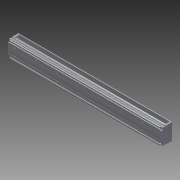
# Autodesk Inventor part: GL15N11060CASW' Body2
Saved by Autodesk Inventor 2011 SP1 (Build 150282100, 282)
## iProperties
Created: 2013-10-24
Part Number: GL15N11060CASW' Body2
Catalog Web Link: www.cadenas.de
Description: Type GL-N-body2-
Vendor: THK
Document SubType Name: Modeling
Designer: PARTuser1
Manufacturer: THK
Density: 1 g/cm^3
Category: PARTsolutions
Company: THK
Title: GL15N11060CASW' Body2
Author: Cadenas PARTsolutions
PSOL_IDENT_0: {$CADENAS_DATA\23d-libs\thk\actuator\type_gl_n\type_gl_n_f_na_1.prj},215 {VTYP=3D},{NB=GL15N11060CAS
PSOL_IDENT_1: W' Body2},{LINA=GL15N11060CASW' Body2},{NN=Type GL-N-body2},{DATE=29.11.2012 11:43:39},{GEOMDATE=29.
PSOL_IDENT_2: 11.2012 11:43:00},{VERSION=},{LINEID=10},{LINESUBID=-1},{WBVAR=L,C,LM,BSE,BSM,LML,BSL}  {NB=GL15N110
PSOL_IDENT_3: 60CASW' Body2},{LINA=GL15N11060CASW' Body2},{KT=DUMMY},{IDNR=},{MN=GL15N},{L=1060},{C=C},{LX=340,460
PSOL_IDENT_4: ,580,700,820,1060,1240,1420},{LM=SW},{VER=1},{DS=Ball screw kit},{BSE=A},{R=15.000},{NDM=2.000},{PCD
PSOL_IDENT_5: =23.000},{BSM=},{BSE1='A','A:inner diameter 30H7,M4,PCD46','B','B:inner diameter 50H7,M5,PCD70','C',
PSOL_IDENT_6: 'C:inner diameter 50H7,M4,PCD60','E','E:inner diameter 30H7,M3,PCD45','F','F:inner diameter 50H7,M4,
PSOL_IDENT_7: PCD70','G','G:inner diameter 34H7,M3,PCD48','H','H:inner diameter 36H7,M4,mounting aperture pitch 50
PSOL_IDENT_8: ','T'  , 'T:inner diameter 22,counter bore for M3 from rear,mounting pitch 31', 'U'  , 'U:inner diam
PSOL_IDENT_9: eter 38.1,M3.mounting pitch 47.14', 'W'  , 'W:inner diameter 40H7 ,M5,PCD63', 'Z'  , 'Z:inner diamet
PSOL_IDENT_10: er 60H7 ,M5,PCD75'},{SD=39},{SD1=27},{TL=126.000},{B=38.000},{TL1=160.000},{B1=45.000},{DS1=Bx},{LML
PSOL_IDENT_11: ='},{BSL=},{BSL1='', 'No mark:Not provided with QZ', 'Q', 'Q:Provided with QZ'},{N=6},{N1=4},{N2=6.0
PSOL_IDENT_12: 00},{N3=4},{BSM1='', 'No:Direct mounting', 'R1', 'R1:Right side motor wrap', 'R2'  , 'R2:Left side m
PSOL_IDENT_13: otor wrap', 'R3', 'R3:Bottom'}
CNS_NB: GL15N11060CASW' Body2
CNS_NBSYN: $MN.$VER.$L.$C.$BSE.$BSM.$LM.$LML.$BSL. Body2
CNS_LINA: GL15N11060CASW' Body2
CNS_MN: GL15N
CNS_L: 1060
CNS_C: Yes
CNS_LX: 340,460,580,700,820,1060,1240,1420
CNS_LM: SSR-XW (L-type table)
CNS_VER: 1
CNS_DS: Ball screw kit
CNS_BSE: A:inner diameter 30H7,M4,PCD46
CNS_R: 15.000
CNS_NDM: 2.000
CNS_PCD: 23.000
CNS_BSM: No:Direct mounting
CNS_BSE1: 'A','A:inner diameter 30H7,M4,PCD46','B','B:inner diameter 50H7,M5,PCD70','C','C:inner diameter 50H7,M4,PCD60','E','E:inner diameter 30H7,M3,PCD45','F','F:inner diameter 50H7,M4,PCD70','G','G:inner diameter 34H7,M3,PCD48','H','H:inner diameter 36H7,M4,mounting aperture pitch 50','T'  , 'T:inner diameter 22,counter bore for M3 from rear,mounting pitch 31', 'U'  , 'U:inner diameter 38.1,M3.mounting pitch 47.14', 'W'  , 'W:inner diameter 40H7 ,M5,PCD63', 'Z'  , 'Z:inner diameter 60H7 ,M5,PCD75'
CNS_SD: 39
CNS_SD1: 27
CNS_TL: 126.000
CNS_B: 38.000
CNS_TL1: 160.000
CNS_B1: 45.000
CNS_DS1: Bx
CNS_LML: No mark:Not provided with QZ
CNS_BSL: No mark:Not provided with QZ
CNS_BSL1: '', 'No mark:Not provided with QZ', 'Q', 'Q:Provided with QZ'
CNS_N: 6.000
CNS_N1: 4.000
CNS_N2: 6.000
CNS_N3: 4.000
CNS_BSM1: '', 'No:Direct mounting', 'R1', 'R1:Right side motor wrap', 'R2'  , 'R2:Left side motor wrap', 'R3', 'R3:Bottom'
SUPPLIER: THK
ARTICLENO: GL15N11060CASW' Body2
BOMINFO: GL15N11060CASW' Body2
CREATOR: CADENAS GmbH
Autodesk Inventor part; units mm, degrees
sketch "Sketch_1" plane through (0, 0, 0) normal (1, 0, 0) x (0, 1, 0)
  line L0 (18.1, 58) -> (12.47, 58)
  arc A0 (12.47, 58) -> (12, 57.53) centre (12.47, 57.53) ccw
  line L1 (12, 57.53) -> (12, 54.97)
  arc A1 (11.53, 54.5) -> (12, 54.97) centre (11.53, 54.97) ccw
  line L2 (11.53, 54.5) -> (6.47, 54.5)
  arc A2 (6, 54.97) -> (6.47, 54.5) centre (6.47, 54.97) ccw
  line L3 (6, 54.97) -> (6, 57.53)
  arc A3 (6, 57.53) -> (5.53, 58) centre (5.53, 57.53) ccw
  line L4 (5.53, 58) -> (3.14, 58)
  arc A4 (3.14, 58) -> (0, 54.86) centre (3.14, 54.86) ccw
  line L5 (0, 54.86) -> (0, 48.5)
  arc A5 (0, 48.5) -> (0.5, 48) centre (0.5, 48.5) ccw
  line L6 (0.5, 48) -> (3.5, 48)
  arc A6 (3.5, 48) -> (4, 48.5) centre (3.5, 48.5) ccw
  line L7 (4, 48.5) -> (4, 50)
  arc A7 (4.5, 50.5) -> (4, 50) centre (4.5, 50) ccw
  line L8 (4.5, 50.5) -> (8.5, 50.5)
  arc A8 (9, 50) -> (8.5, 50.5) centre (8.5, 50) ccw
  line L9 (9, 50) -> (9, 48.8)
  arc A9 (9, 48.8) -> (9.3, 48.5) centre (9.3, 48.8) ccw
  line L10 (9.3, 48.5) -> (9.7, 48.5)
  arc A10 (10, 48.2) -> (9.7, 48.5) centre (9.7, 48.2) ccw
  line L11 (10, 48.2) -> (10, 41.8)
  arc A11 (9.7, 41.5) -> (10, 41.8) centre (9.7, 41.8) ccw
  line L12 (9.7, 41.5) -> (9.3, 41.5)
  arc A12 (9.3, 41.5) -> (9, 41.2) centre (9.3, 41.2) ccw
  line L13 (9, 41.2) -> (9, 40)
  arc A13 (8.5, 39.5) -> (9, 40) centre (8.5, 40) ccw
  line L14 (8.5, 39.5) -> (4.5, 39.5)
  arc A14 (4, 40) -> (4.5, 39.5) centre (4.5, 40) ccw
  line L15 (4, 40) -> (4, 41.5)
  arc A15 (4, 41.5) -> (3.5, 42) centre (3.5, 41.5) ccw
  line L16 (3.5, 42) -> (0.5, 42)
  arc A16 (0.5, 42) -> (0, 41.5) centre (0.5, 41.5) ccw
  line L17 (0, 41.5) -> (0, 24)
  line L18 (0, 24) -> (0.531, 22.938)
  arc A17 (0.635, 22.4347) -> (0.531, 22.938) centre (-0.3634, 22.4908) ccw
  arc A18 (0.635, 22.4347) -> (0.635, -22.4347) centre (400.0054, 0) ccw
  arc A19 (0.531, -22.938) -> (0.635, -22.4347) centre (-0.3634, -22.4908) ccw
  line L19 (0.531, -22.938) -> (0, -24)
  line L20 (0, -24) -> (0, -41.5)
  arc A20 (0, -41.5) -> (0.5, -42) centre (0.5, -41.5) ccw
  line L21 (0.5, -42) -> (3.5, -42)
  arc A21 (3.5, -42) -> (4, -41.5) centre (3.5, -41.5) ccw
  line L22 (4, -41.5) -> (4, -40)
  arc A22 (4.5, -39.5) -> (4, -40) centre (4.5, -40) ccw
  line L23 (4.5, -39.5) -> (8.5, -39.5)
  arc A23 (9, -40) -> (8.5, -39.5) centre (8.5, -40) ccw
  line L24 (9, -40) -> (9, -41.2)
  arc A24 (9, -41.2) -> (9.3, -41.5) centre (9.3, -41.2) ccw
  line L25 (9.3, -41.5) -> (9.7, -41.5)
  arc A25 (10, -41.8) -> (9.7, -41.5) centre (9.7, -41.8) ccw
  line L26 (10, -41.8) -> (10, -48.2)
  arc A26 (9.7, -48.5) -> (10, -48.2) centre (9.7, -48.2) ccw
  line L27 (9.7, -48.5) -> (9.3, -48.5)
  arc A27 (9.3, -48.5) -> (9, -48.8) centre (9.3, -48.8) ccw
  line L28 (9, -48.8) -> (9, -50)
  arc A28 (8.5, -50.5) -> (9, -50) centre (8.5, -50) ccw
  line L29 (8.5, -50.5) -> (4.5, -50.5)
  arc A29 (4, -50) -> (4.5, -50.5) centre (4.5, -50) ccw
  line L30 (4, -50) -> (4, -48.5)
  arc A30 (4, -48.5) -> (3.5, -48) centre (3.5, -48.5) ccw
  line L31 (3.5, -48) -> (0.5, -48)
  arc A31 (0.5, -48) -> (0, -48.5) centre (0.5, -48.5) ccw
  line L32 (0, -48.5) -> (0, -54.86)
  arc A32 (0, -54.86) -> (3.14, -58) centre (3.14, -54.86) ccw
  line L33 (3.14, -58) -> (5.53, -58)
  arc A33 (5.53, -58) -> (6, -57.53) centre (5.53, -57.53) ccw
  line L34 (6, -57.53) -> (6, -54.97)
  arc A34 (6.47, -54.5) -> (6, -54.97) centre (6.47, -54.97) ccw
  line L35 (6.47, -54.5) -> (11.53, -54.5)
  arc A35 (12, -54.97) -> (11.53, -54.5) centre (11.53, -54.97) ccw
  line L36 (12, -54.97) -> (12, -57.53)
  arc A36 (12, -57.53) -> (12.47, -58) centre (12.47, -57.53) ccw
  line L37 (12.47, -58) -> (18.1, -58)
  line L38 (18.1, -58) -> (18.1, -57)
  line L39 (18.1, -57) -> (20.98, -57)
  arc A37 (20.98, -57) -> (21.45, -56.53) centre (20.98, -56.53) ccw
  line L40 (21.45, -56.53) -> (21.45, -55.97)
  arc A38 (21.45, -55.97) -> (20.98, -55.5) centre (20.98, -55.97) ccw
  line L41 (20.98, -55.5) -> (20.9, -55.5)
  arc A39 (20.7, -55.3) -> (20.9, -55.5) centre (20.9, -55.3) ccw
  line L42 (20.7, -55.3) -> (20.7, -53.3)
  arc A40 (21, -53) -> (20.7, -53.3) centre (21, -53.3) ccw
  line L43 (21, -53) -> (22, -53)
  arc A41 (22, -53) -> (22.2, -52.8) centre (22, -52.8) ccw
  arc A42 (22.5, -52.5) -> (22.2, -52.8) centre (22.5, -52.8) ccw
  line L44 (22.5, -52.5) -> (24.7, -52.5)
  arc A43 (25, -52.8) -> (24.7, -52.5) centre (24.7, -52.8) ccw
  arc A44 (25, -52.8) -> (25.2, -53) centre (25.2, -52.8) ccw
  line L45 (25.2, -53) -> (26.2, -53)
  arc A45 (26.5, -53.3) -> (26.2, -53) centre (26.2, -53.3) ccw
  line L46 (26.5, -53.3) -> (26.5, -55.3)
  arc A46 (26.3, -55.5) -> (26.5, -55.3) centre (26.3, -55.3) ccw
  line L47 (26.3, -55.5) -> (26.22, -55.5)
  arc A47 (26.22, -55.5) -> (25.75, -55.97) centre (26.22, -55.97) ccw
  line L48 (25.75, -55.97) -> (25.75, -56.53)
  arc A48 (25.75, -56.53) -> (26.22, -57) centre (26.22, -56.53) ccw
  line L49 (26.22, -57) -> (29.1, -57)
  line L50 (29.1, -57) -> (29.1, -58)
  line L51 (29.1, -58) -> (31.6, -58)
  line L52 (31.6, -58) -> (33, -56.6)
  line L53 (33, -56.6) -> (33, -52.5)
  line L54 (33, -52.5) -> (34.32, -52.5)
  line L55 (34.32, -52.5) -> (37.42, -49.4)
  line L56 (37.42, -49.4) -> (40.4, -49.4)
  line L57 (40.4, -49.4) -> (43.5, -52.5)
  line L58 (43.5, -52.5) -> (44.8, -52.5)
  line L59 (44.8, -52.5) -> (45.6, -51.7)
  line L60 (45.6, -51.7) -> (45.6, -38.3)
  line L61 (45.6, -38.3) -> (44.8, -37.5)
  line L62 (44.8, -37.5) -> (43.5, -37.5)
  line L63 (43.5, -37.5) -> (40.37, -40.63)
  line L64 (40.37, -40.63) -> (37.45, -40.63)
  line L65 (37.45, -40.63) -> (34.32, -37.5)
  line L66 (34.32, -37.5) -> (32.2, -37.5)
  line L67 (32.2, -37.5) -> (32.2, -33.5)
  arc A49 (32.2, -33.5) -> (31.7, -33) centre (31.7, -33.5) ccw
  line L68 (31.7, -33) -> (17, -33)
  arc A50 (16, -32) -> (17, -33) centre (17, -32) ccw
  line L69 (16, -32) -> (16, 32)
  arc A51 (17, 33) -> (16, 32) centre (17, 32) ccw
  line L70 (17, 33) -> (31.7, 33)
  arc A52 (31.7, 33) -> (32.2, 33.5) centre (31.7, 33.5) ccw
  line L71 (32.2, 33.5) -> (32.2, 37.5)
  line L72 (32.2, 37.5) -> (34.32, 37.5)
  line L73 (34.32, 37.5) -> (37.45, 40.63)
  line L74 (37.45, 40.63) -> (40.37, 40.63)
  line L75 (40.37, 40.63) -> (43.5, 37.5)
  line L76 (43.5, 37.5) -> (44.8, 37.5)
  line L77 (44.8, 37.5) -> (45.6, 38.3)
  line L78 (45.6, 38.3) -> (45.6, 51.7)
  line L79 (45.6, 51.7) -> (44.8, 52.5)
  line L80 (44.8, 52.5) -> (43.5, 52.5)
  line L81 (43.5, 52.5) -> (40.4, 49.4)
  line L82 (40.4, 49.4) -> (37.42, 49.4)
  line L83 (37.42, 49.4) -> (34.32, 52.5)
  line L84 (34.32, 52.5) -> (33, 52.5)
  line L85 (33, 52.5) -> (33, 56.6)
  line L86 (33, 56.6) -> (31.6, 58)
  line L87 (31.6, 58) -> (29.1, 58)
  line L88 (29.1, 58) -> (29.1, 57)
  line L89 (29.1, 57) -> (26.22, 57)
  arc A53 (26.22, 57) -> (25.75, 56.53) centre (26.22, 56.53) ccw
  line L90 (25.75, 56.53) -> (25.75, 55.97)
  arc A54 (25.75, 55.97) -> (26.22, 55.5) centre (26.22, 55.97) ccw
  line L91 (26.22, 55.5) -> (26.3, 55.5)
  arc A55 (26.5, 55.3) -> (26.3, 55.5) centre (26.3, 55.3) ccw
  line L92 (26.5, 55.3) -> (26.5, 53.3)
  arc A56 (26.2, 53) -> (26.5, 53.3) centre (26.2, 53.3) ccw
  line L93 (26.2, 53) -> (25.2, 53)
  arc A57 (25.2, 53) -> (25, 52.8) centre (25.2, 52.8) ccw
  arc A58 (24.7, 52.5) -> (25, 52.8) centre (24.7, 52.8) ccw
  line L94 (24.7, 52.5) -> (22.5, 52.5)
  arc A59 (22.2, 52.8) -> (22.5, 52.5) centre (22.5, 52.8) ccw
  arc A60 (22.2, 52.8) -> (22, 53) centre (22, 52.8) ccw
  line L95 (22, 53) -> (21, 53)
  arc A61 (20.7, 53.3) -> (21, 53) centre (21, 53.3) ccw
  line L96 (20.7, 53.3) -> (20.7, 55.3)
  arc A62 (20.9, 55.5) -> (20.7, 55.3) centre (20.9, 55.3) ccw
  line L97 (20.9, 55.5) -> (20.98, 55.5)
  arc A63 (20.98, 55.5) -> (21.45, 55.97) centre (20.98, 55.97) ccw
  line L98 (21.45, 55.97) -> (21.45, 56.53)
  arc A64 (21.45, 56.53) -> (20.98, 57) centre (20.98, 56.53) ccw
  line L99 (20.98, 57) -> (18.1, 57)
  line L100 (18.1, 57) -> (18.1, 58)
  constraints: 202 end point, 130 point on circle, 65 centre point
extrude "Extrusion1" add sketch "Sketch_1" along normal blind 1060
sketch "Sketch_2" plane through (0, 0, 0) normal (1, 0, 0) x (0, 1, 0)
  line L0 (68.3, 57) -> (27.6, 57)
  line L1 (27.6, 57) -> (27.6, 53)
  line L2 (27.6, 53) -> (19.6, 53)
  line L3 (19.6, 53) -> (19.6, 57)
  line L4 (19.6, 57) -> (12.12, 57)
  line L5 (12.12, 57) -> (10, 54.88)
  line L6 (10, 54.88) -> (10, 38.5)
  line L7 (10, 38.5) -> (3.41, 38.5)
  line L8 (3.41, 38.5) -> (2, 37.09)
  line L9 (2, 37.09) -> (2, -37.09)
  line L10 (2, -37.09) -> (3.41, -38.5)
  line L11 (3.41, -38.5) -> (10, -38.5)
  line L12 (10, -38.5) -> (10, -54.88)
  line L13 (10, -54.88) -> (12.12, -57)
  line L14 (12.12, -57) -> (19.6, -57)
  line L15 (19.6, -57) -> (19.6, -53)
  line L16 (19.6, -53) -> (27.6, -53)
  line L17 (27.6, -53) -> (27.6, -57)
  line L18 (27.6, -57) -> (68.3, -57)
  line L19 (68.3, -57) -> (68.3, -50)
  line L20 (68.3, -50) -> (72.3, -50)
  line L21 (72.3, -50) -> (72.3, 50)
  line L22 (72.3, 50) -> (68.3, 50)
  line L23 (68.3, 50) -> (68.3, 57)
  constraints: 48 end point
extrude "Extrusion2" add sketch "Sketch_2" against normal blind 12
sketch "Sketch_3" plane through (1060, 0, 0) normal (1, 0, 0) x (0, 0, -1)
  line L0 (-57, 68.3) -> (-57, 27.6)
  line L1 (-57, 27.6) -> (-53, 27.6)
  line L2 (-53, 27.6) -> (-53, 19.6)
  line L3 (-53, 19.6) -> (-57, 19.6)
  line L4 (-57, 19.6) -> (-57, 12.12)
  line L5 (-57, 12.12) -> (-54.88, 10)
  line L6 (-54.88, 10) -> (-38.5, 10)
  line L7 (-38.5, 10) -> (-38.5, 3.41)
  line L8 (-38.5, 3.41) -> (-37.09, 2)
  line L9 (-37.09, 2) -> (37.09, 2)
  line L10 (37.09, 2) -> (38.5, 3.41)
  line L11 (38.5, 3.41) -> (38.5, 10)
  line L12 (38.5, 10) -> (54.88, 10)
  line L13 (54.88, 10) -> (57, 12.12)
  line L14 (57, 12.12) -> (57, 19.6)
  line L15 (57, 19.6) -> (53, 19.6)
  line L16 (53, 19.6) -> (53, 27.6)
  line L17 (53, 27.6) -> (57, 27.6)
  line L18 (57, 27.6) -> (57, 68.3)
  line L19 (57, 68.3) -> (50, 68.3)
  line L20 (50, 68.3) -> (50, 72.3)
  line L21 (50, 72.3) -> (-50, 72.3)
  line L22 (-50, 72.3) -> (-50, 68.3)
  line L23 (-50, 68.3) -> (-57, 68.3)
  constraints: 48 end point
extrude "Extrusion3" add sketch "Sketch_3" along normal blind 12
sketch "Sketch_4" plane through (54.5, 0, 0) normal (1, 0, 0) x (0, 0, -1)
  line L0 (-30, 47.1) -> (-30, 17.4)
  line L1 (-30, 17.4) -> (-28.6, 16)
  line L2 (-28.6, 16) -> (28.6, 16)
  line L3 (28.6, 16) -> (30, 17.4)
  line L4 (30, 17.4) -> (30, 47.1)
  line L5 (30, 47.1) -> (28.6, 48.5)
  line L6 (28.6, 48.5) -> (17, 48.5)
  line L7 (17, 48.5) -> (17, 53)
  line L8 (17, 53) -> (15, 55)
  line L9 (15, 55) -> (-15, 55)
  line L10 (-15, 55) -> (-17, 53)
  line L11 (-17, 53) -> (-17, 48.5)
  line L12 (-17, 48.5) -> (-28.6, 48.5)
  line L13 (-28.6, 48.5) -> (-30, 47.1)
  constraints: 28 end point
extrude "Extrusion4" add sketch "Sketch_4" along normal blind 24
sketch "Sketch_5" plane through (1060, 0, 0) normal (1, 0, 0) x (0, 0, -1)
  line L0 (-30, 47.1) -> (-30, 17.4)
  line L1 (-30, 17.4) -> (-28.6, 16)
  line L2 (-28.6, 16) -> (28.6, 16)
  line L3 (28.6, 16) -> (30, 17.4)
  line L4 (30, 17.4) -> (30, 47.1)
  line L5 (30, 47.1) -> (28.6, 48.5)
  line L6 (28.6, 48.5) -> (17, 48.5)
  line L7 (17, 48.5) -> (17, 53)
  line L8 (17, 53) -> (15, 55)
  line L9 (15, 55) -> (-15, 55)
  line L10 (-15, 55) -> (-17, 53)
  line L11 (-17, 53) -> (-17, 48.5)
  line L12 (-17, 48.5) -> (-28.6, 48.5)
  line L13 (-28.6, 48.5) -> (-30, 47.1)
  constraints: 28 end point
extrude "Extrusion5" add sketch "Sketch_5" against normal blind 20
sketch "Sketch6" plane through (78.5, 0, 0) normal (1, 0, 0) x (0, 0, -1)
  point P0 (0, 38)
hole "Drilling 1" at (78.5, 38, 0) direction (-1, 0, 0) diameter 14 depth 4.5
sketch "Sketch7" plane through (0, 0, 0) normal (1, 0, 0) x (0, 0, -1)
  point P0 (0, 38)
hole "Drilling 2" at (0, 38, 0) direction (-1, 0, 0) diameter 30 depth 12
sketch "Sketch8" plane through (0, 0, 0) normal (1, 0, 0) x (0, 0, -1)
  point P0 (-16.2635, 21.7365)
hole "Drilling 3" at (0, 21.7365, 16.2635) direction (-1, 0, 0) diameter 3.242 depth 12 countersink diameter 4 countersink angle 90 thread size "M4x0.7" class "6H" standard "ISO Metric profile"
sketch "Sketch9" plane through (0, 0, 0) normal (1, 0, 0) x (0, 0, -1)
  point P0 (16.2635, 54.2635)
hole "Drilling 4" at (0, 54.2635, -16.2635) direction (-1, 0, 0) diameter 3.242 depth 12 countersink diameter 4 countersink angle 90 thread size "M4x0.7" class "6H" standard "ISO Metric profile"
sketch "Sketch10" plane through (0, 0, 0) normal (1, 0, 0) x (0, 0, -1)
  point P0 (-16.2635, 54.2635)
hole "Drilling 5" at (0, 54.2635, 16.2635) direction (-1, 0, 0) diameter 3.242 depth 12 countersink diameter 4 countersink angle 90 thread size "M4x0.7" class "6H" standard "ISO Metric profile"
sketch "Sketch11" plane through (0, 0, 0) normal (1, 0, 0) x (0, 0, -1)
  point P0 (16.2635, 21.7365)
hole "Drilling 6" at (0, 21.7365, -16.2635) direction (-1, 0, 0) diameter 3.242 depth 12 countersink diameter 4 countersink angle 90 thread size "M4x0.7" class "6H" standard "ISO Metric profile"
sketch "Sketch12" plane through (1040, 0, 0) normal (-1, 0, 0) x (0, 0, 1)
  point P0 (0, 38)
hole "Drilling 7" at (1040, 38, 0) direction (1, 0, 0) diameter 22 depth 5.7
sketch "Sketch_18" plane through (0, 0, 0) normal (0, 0, 1) x (1, 0, 0)
  line L0 (50, 38) -> (-50, 38)
  line L1 (54.5, 48.5) -> (77, 48.5)
  line L2 (77, 48.5) -> (77, 49)
  line L3 (77, 49) -> (54.5, 49)
  line L4 (54.5, 49) -> (54.5, 48.5)
  constraints: 10 end point
revolve "Revolution1" cut sketch "Sketch_18" angle 360 about axis through (50, 38, 0) along (1, 0, 0)
sketch "Sketch_15" plane through (0, 0, 0) normal (0, 0, 1) x (1, 0, 0)
  line L0 (1044.8, 38) -> (72.8, 38)
  line L1 (72.8, 38) -> (72.8, 44)
  line L2 (72.8, 44) -> (78.6, 44)
  line L3 (78.6, 44) -> (78.6, 45.2)
  line L4 (78.6, 45.2) -> (79.4, 46)
  line L5 (79.4, 46) -> (1044, 46)
  line L6 (1044, 46) -> (1044.8, 45.2)
  line L7 (1044.8, 45.2) -> (1044.8, 38)
  line L8 (1044.8, 38) -> (72.8, 38)
  constraints: 18 end point
revolve "Revolution2" add sketch "Sketch_15" angle 360 about axis through (1044.8, 38, 0) along (1, 0, 0)
sketch "Sketch_19" plane through (54.5, 0, 0) normal (1, 0, 0) x (0, 0, -1)
  line L0 (-17, 50) -> (-17, 26)
  line L1 (-17, 26) -> (-12, 21)
  line L2 (-12, 21) -> (12, 21)
  line L3 (12, 21) -> (17, 26)
  line L4 (17, 26) -> (17, 50)
  line L5 (17, 50) -> (12, 55)
  line L6 (12, 55) -> (-12, 55)
  line L7 (-12, 55) -> (-17, 50)
  constraints: 16 end point
extrude "Extrusion6" add sketch "Sketch_19" against normal blind 5
sketch "Sketch16" plane through (49.5, 0, 0) normal (-1, 0, 0) x (0, 0, 1)
  point P0 (0, 38)
hole "Drilling 8" at (49.5, 38, 0) direction (1, 0, 0) diameter 21 depth 3.25 countersink diameter 24 countersink angle 112.62
sketch "Sketch_21" plane through (52.75, 0, 0) normal (1, 0, 0) x (0, 0, -1)
  line L0 (-9.1924, 40.1213) -> (-9.1924, 35.8787)
  line L1 (-9.1924, 35.8787) -> (-2.1213, 28.8076)
  line L2 (-2.1213, 28.8076) -> (2.1213, 28.8076)
  line L3 (2.1213, 28.8076) -> (9.1924, 35.8787)
  line L4 (9.1924, 35.8787) -> (9.1924, 40.1213)
  line L5 (9.1924, 40.1213) -> (2.1213, 47.1924)
  line L6 (2.1213, 47.1924) -> (-2.1213, 47.1924)
  line L7 (-2.1213, 47.1924) -> (-9.1924, 40.1213)
  constraints: 16 end point
extrude "Extrusion7" add sketch "Sketch_21" against normal blind 7.75
sketch "Sketch_22" plane through (85, 0, 0) normal (1, 0, 0) x (0, 0, -1)
  line L0 (-8, 30) -> (-6, 30)
  line L1 (-6, 30) -> (-6, 46)
  line L2 (-6, 46) -> (-8, 46)
  line L3 (-8, 46) -> (-8, 30)
  constraints: 8 end point
extrude "Extrusion8" cut sketch "Sketch_22" along normal blind 8
sketch "Sketch_23" plane through (85, 0, 0) normal (1, 0, 0) x (0, 0, -1)
  line L0 (6, 30) -> (8, 30)
  line L1 (8, 30) -> (8, 46)
  line L2 (8, 46) -> (6, 46)
  line L3 (6, 46) -> (6, 30)
  constraints: 8 end point
extrude "Extrusion9" cut sketch "Sketch_23" along normal blind 8
sketch "Sketch_24" plane through (0, 0, 0) normal (0, 0, 1) x (1, 0, 0)
  line L0 (45, 38) -> (25, 38)
  line L1 (25, 38) -> (25, 41.6)
  line L2 (25, 41.6) -> (25.4, 42)
  line L3 (25.4, 42) -> (40, 42)
  line L4 (40, 42) -> (40, 42.5)
  line L5 (40, 42.5) -> (40.5, 43)
  line L6 (40.5, 43) -> (45, 43)
  line L7 (45, 43) -> (45, 38)
  line L8 (45, 38) -> (25, 38)
  constraints: 18 end point
revolve "Revolution3" add sketch "Sketch_24" angle 360 about axis through (45, 38, 0) along (1, 0, 0)
sketch "Sketch_25" plane through (60.5, 0, 0) normal (1, 0, 0) x (0, 0, -1)
  line L0 (23, 49.5) -> (23, 48.5)
  line L1 (23, 48.5) -> (18, 48.5)
  line L2 (18, 48.5) -> (18, 49.5)
  line L3 (18, 49.5) -> (23, 49.5)
  line L4 (23, 49.5) -> (23, 48.5)
  constraints: 10 end point
revolve "Revolution4" add sketch "Sketch_25" angle 360 about axis through (60.5, 49.5, -23) along (0, 1, 0)
sketch "Sketch_26" plane through (60.5, 0, 0) normal (1, 0, 0) x (0, 0, -1)
  line L0 (-23, 48.5) -> (-23, 49.5)
  line L1 (-23, 49.5) -> (-18, 49.5)
  line L2 (-18, 49.5) -> (-18, 48.5)
  line L3 (-18, 48.5) -> (-23, 48.5)
  line L4 (-23, 48.5) -> (-23, 49.5)
  constraints: 10 end point
revolve "Revolution5" add sketch "Sketch_26" angle 360 about axis through (60.5, 48.5, 23) along (0, -1, 0)
sketch "Sketch_27" plane through (72.5, 0, 0) normal (1, 0, 0) x (0, 0, -1)
  line L0 (23, 49.5) -> (23, 48.5)
  line L1 (23, 48.5) -> (18, 48.5)
  line L2 (18, 48.5) -> (18, 49.5)
  line L3 (18, 49.5) -> (23, 49.5)
  line L4 (23, 49.5) -> (23, 48.5)
  constraints: 10 end point
revolve "Revolution6" add sketch "Sketch_27" angle 360 about axis through (72.5, 49.5, -23) along (0, 1, 0)
sketch "Sketch_28" plane through (72.5, 0, 0) normal (1, 0, 0) x (0, 0, -1)
  line L0 (-23, 49.5) -> (-23, 48.5)
  line L1 (-23, 48.5) -> (-28, 48.5)
  line L2 (-28, 48.5) -> (-28, 49.5)
  line L3 (-28, 49.5) -> (-23, 49.5)
  line L4 (-23, 49.5) -> (-23, 48.5)
  constraints: 10 end point
revolve "Revolution7" add sketch "Sketch_28" angle 360 about axis through (72.5, 49.5, 23) along (0, 1, 0)
sketch "Sketch_29" plane through (1050, 0, 0) normal (1, 0, 0) x (0, 0, -1)
  line L0 (23, 49.5) -> (23, 48.5)
  line L1 (23, 48.5) -> (18, 48.5)
  line L2 (18, 48.5) -> (18, 49.5)
  line L3 (18, 49.5) -> (23, 49.5)
  line L4 (23, 49.5) -> (23, 48.5)
  constraints: 10 end point
revolve "Revolution8" add sketch "Sketch_29" angle 360 about axis through (1050, 49.5, -23) along (0, 1, 0)
sketch "Sketch_30" plane through (1050, 0, 0) normal (1, 0, 0) x (0, 0, -1)
  line L0 (-23, 49.5) -> (-23, 48.5)
  line L1 (-23, 48.5) -> (-28, 48.5)
  line L2 (-28, 48.5) -> (-28, 49.5)
  line L3 (-28, 49.5) -> (-23, 49.5)
  line L4 (-23, 49.5) -> (-23, 48.5)
  constraints: 10 end point
revolve "Revolution9" add sketch "Sketch_30" angle 360 about axis through (1050, 49.5, 23) along (0, 1, 0)
sketch "Sketch27" plane through (1072, 0, 0) normal (1, 0, 0) x (0, 0, -1)
  point P0 (38, 64.5)
hole "Drilling 9" at (1072, 64.5, -38) direction (-1, 0, 0) diameter 4.134 depth 12 countersink diameter 5 countersink angle 90 thread size "M5x0.8" class "6H" standard "ISO Metric profile"
sketch "Sketch_33" plane through (1060, 0, 0) normal (1, 0, 0) x (0, 0, -1)
  line L0 (34, 66.8094) -> (34, 62.1906)
  line L1 (34, 62.1906) -> (38, 59.8812)
  line L2 (38, 59.8812) -> (42, 62.1906)
  line L3 (42, 62.1906) -> (42, 66.8094)
  line L4 (42, 66.8094) -> (38, 69.1188)
  line L5 (38, 69.1188) -> (34, 66.8094)
  constraints: 12 end point
extrude "Extrusion10" add sketch "Sketch_33" against normal blind 3.2
sketch "Sketch_34" plane through (0, 0, -38) normal (0, 0, 1) x (1, 0, 0)
  line L0 (1056.8, 64.5) -> (1035, 64.5)
  line L1 (1035, 64.5) -> (1035, 70.75)
  line L2 (1035, 70.75) -> (1044, 70.75)
  line L3 (1044, 70.75) -> (1044, 67)
  line L4 (1044, 67) -> (1056.8, 67)
  line L5 (1056.8, 67) -> (1056.8, 64.5)
  line L6 (1056.8, 64.5) -> (1035, 64.5)
  constraints: 14 end point
revolve "Revolution10" add sketch "Sketch_34" angle 360 about axis through (1056.8, 64.5, -38) along (1, 0, 0)
sketch "Sketch_35" plane through (-12, 0, 0) normal (1, 0, 0) x (0, 0, -1)
  line L0 (-59, 72.54) -> (-59, 69.56)
  arc A0 (-59, 69.56) -> (-57.74, 68.3) centre (-57.74, 69.56) ccw
  line L1 (-57.74, 68.3) -> (-51, 68.3)
  line L2 (-51, 68.3) -> (-51, 69.8)
  line L3 (-51, 69.8) -> (-57.5, 69.8)
  line L4 (-57.5, 69.8) -> (-57.5, 72.3)
  line L5 (-57.5, 72.3) -> (57.5, 72.3)
  line L6 (57.5, 72.3) -> (57.5, 69.8)
  line L7 (57.5, 69.8) -> (51, 69.8)
  line L8 (51, 69.8) -> (51, 68.3)
  line L9 (51, 68.3) -> (57.74, 68.3)
  arc A1 (57.74, 68.3) -> (59, 69.56) centre (57.74, 69.56) ccw
  line L10 (59, 69.56) -> (59, 72.54)
  arc A2 (59, 72.54) -> (57.74, 73.8) centre (57.74, 72.54) ccw
  line L11 (57.74, 73.8) -> (-57.74, 73.8)
  arc A3 (-57.74, 73.8) -> (-59, 72.54) centre (-57.74, 72.54) ccw
  constraints: 24 end point, 8 point on circle, 4 centre point
extrude "Extrusion11" add sketch "Sketch_35" along normal blind 1084
sketch "Sketch_36" plane through (0, 0, 32) normal (0, 0, 1) x (1, 0, 0)
  line L0 (-6, 73.8) -> (-6, 75)
  line L1 (-6, 75) -> (-2, 75)
  line L2 (-2, 75) -> (-2, 73.8)
  line L3 (-2, 73.8) -> (-6, 73.8)
  line L4 (-6, 73.8) -> (-6, 75)
  constraints: 10 end point
revolve "Revolution11" add sketch "Sketch_36" angle 360 about axis through (-6, 73.8, 32) along (0, -1, 0)
sketch "Sketch_37" plane through (0, 0, 32) normal (0, 0, 1) x (1, 0, 0)
  line L0 (1066, 73.8) -> (1066, 75)
  line L1 (1066, 75) -> (1070, 75)
  line L2 (1070, 75) -> (1070, 73.8)
  line L3 (1070, 73.8) -> (1066, 73.8)
  line L4 (1066, 73.8) -> (1066, 75)
  constraints: 10 end point
revolve "Revolution12" add sketch "Sketch_37" angle 360 about axis through (1066, 73.8, 32) along (0, -1, 0)
sketch "Sketch_38" plane through (0, 0, -32) normal (0, 0, 1) x (1, 0, 0)
  line L0 (-6, 73.8) -> (-6, 75)
  line L1 (-6, 75) -> (-2, 75)
  line L2 (-2, 75) -> (-2, 73.8)
  line L3 (-2, 73.8) -> (-6, 73.8)
  line L4 (-6, 73.8) -> (-6, 75)
  constraints: 10 end point
revolve "Revolution13" add sketch "Sketch_38" angle 360 about axis through (-6, 73.8, -32) along (0, -1, 0)
sketch "Sketch_39" plane through (0, 0, -32) normal (0, 0, 1) x (1, 0, 0)
  line L0 (1066, 73.8) -> (1066, 75)
  line L1 (1066, 75) -> (1070, 75)
  line L2 (1070, 75) -> (1070, 73.8)
  line L3 (1070, 73.8) -> (1066, 73.8)
  line L4 (1066, 73.8) -> (1066, 75)
  constraints: 10 end point
revolve "Revolution14" add sketch "Sketch_39" angle 360 about axis through (1066, 73.8, -32) along (0, -1, 0)
sketch "Sketch35" plane through (0, 16, 32) normal (0, 1, 0) x (1, 0, 0)
  point P0 (35, 57)
hole "Drilling 10" at (35, 16, -25) direction (0, -1, 0) diameter 6.6 depth 16 counterbore diameter 11 counterbore depth 11
sketch "Sketch36" plane through (0, 16, 32) normal (0, 1, 0) x (1, 0, 0)
  point P0 (35, 7)
hole "Drilling 11" at (35, 16, 25) direction (0, -1, 0) diameter 6.6 depth 16 counterbore diameter 11 counterbore depth 11
pattern_linear "Rectangular Pattern1" count 7 spacing 150 along (1, 0, 0) of "Drilling 11"
pattern_linear "Rectangular Pattern2" count 7 spacing 150 along (1, 0, 0) of "Drilling 10"
ref_plane "type_gl_n_bt_XY" through (39, 38, 0) normal (-1, 0, 0) x (0, 0, -1)
ref_plane "type_gl_n_bt_YZ" through (39, 38, 0) normal (0, 0, -1) x (0, -1, 0)
ref_plane "type_gl_n_bt_ZX" through (39, 38, 0) normal (0, -1, 0) x (-1, 0, 0)
ref_plane "type_gl_n_bx_XY" through (-12, 38, 0) normal (1, 0, 0) x (0, 0, -1)
ref_plane "type_gl_n_bx_YZ" through (-12, 38, 0) normal (0, 0, -1) x (0, 1, 0)
ref_plane "type_gl_n_bx_ZX" through (-12, 38, 0) normal (0, 1, 0) x (1, 0, 0)
ref_plane "type_gl_n_dummy1_XY" through (0, 0, 0) normal (0, 1, 0) x (1, 0, 0)
ref_plane "type_gl_n_dummy1_YZ" through (0, 0, 0) normal (1, 0, 0) x (0, 0, -1)
ref_plane "type_gl_n_dummy1_ZX" through (0, 0, 0) normal (0, 0, -1) x (0, 1, 0)
ref_plane "type_gl_n_s1_XY" through (78.5, 23.6, 53) normal (0, 0, -1) x (1, 0, 0)
ref_plane "type_gl_n_s1_YZ" through (78.5, 23.6, 53) normal (1, 0, 0) x (0, -1, 0)
ref_plane "type_gl_n_s1_ZX" through (78.5, 23.6, 53) normal (0, -1, 0) x (0, 0, -1)
ref_plane "type_gl_n_s2_XY" through (511, 23.6, 53) normal (0, 0, -1) x (1, 0, 0)
ref_plane "type_gl_n_s2_YZ" through (511, 23.6, 53) normal (1, 0, 0) x (0, -1, 0)
ref_plane "type_gl_n_s2_ZX" through (511, 23.6, 53) normal (0, -1, 0) x (0, 0, -1)
ref_plane "type_gl_n_s3_XY" through (943.5, 23.6, 53) normal (0, 0, -1) x (1, 0, 0)
ref_plane "type_gl_n_s3_YZ" through (943.5, 23.6, 53) normal (1, 0, 0) x (0, -1, 0)
ref_plane "type_gl_n_s3_ZX" through (943.5, 23.6, 53) normal (0, -1, 0) x (0, 0, -1)
body "Solid1"
